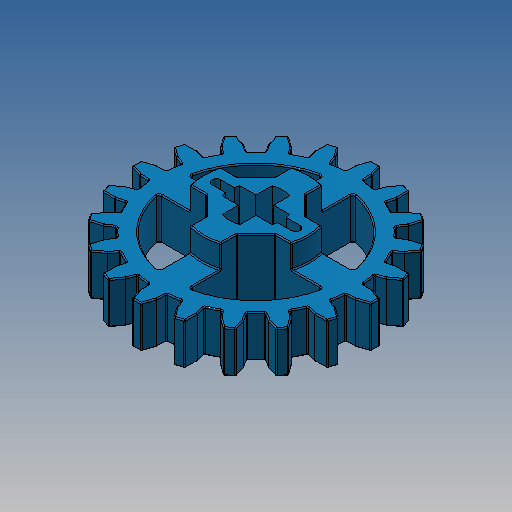
# Autodesk Inventor part: 69779-DkAzure
Saved by Autodesk Inventor 2025 (Build 290162010, 162A)
## iProperties
Created: 2014-08-13
Part Number: 69779-DkAzure
Material: ABS Plastic
Document SubType Name: Modeling
Designer: h.muther
Density: 1.06 g/cm^3
Appearance: DkAzure
Mass: 0.705537 g
Surface Area: 11.2279 cm^2
Volume: 0.665601 cm^3
Description: Technic, Gear 20
Author: h.muther
Autodesk Inventor part; units mm, degrees
ref_plane "YZ Plane" through (0, 0, 0) normal (1, 0, 0) x (0, 1, 0)
ref_plane "XZ Plane" through (0, 0, 0) normal (0, 1, 0) x (-1, 0, 0)
ref_plane "XY Plane" through (0, 0, 0) normal (0, 0, 1) x (1, 0, 0)
sketch "Sketch2" plane through (0, 0, 0) normal (0, 1, 0) x (-1, 0, 0)
  circle A0 centre (0, 0) radius 2.4 construction
  circle A1 centre (0, 0) radius 8.9654
  circle A2 centre (0, 0) radius 7.5654 construction
  circle A3 centre (0, 0) radius 4.8 construction
  circle A4 centre (0, 0) radius 3.6 construction
  line L0 (-0.8, 2.2627) -> (-0.8, 0.8)
  line L1 (-0.8, 0.8) -> (-2.2627, 0.8)
  line L2 (-2.2627, -0.8) -> (-0.8, -0.8)
  line L3 (-0.8, -0.8) -> (-0.8, -2.2627)
  line L4 (0.8, -2.2627) -> (0.8, -0.8)
  line L5 (0.8, -0.8) -> (2.2627, -0.8)
  line L6 (2.2627, 0.8) -> (0.8, 0.8)
  line L7 (0.8, 0.8) -> (0.8, 2.2627)
  arc A5 (0.8, 2.2627) -> (-0.8, 2.2627) centre (0, 0) ccw
  arc A6 (-2.2627, 0.8) -> (-2.2627, -0.8) centre (0, 0) ccw
  arc A7 (-0.8, -2.2627) -> (0.8, -2.2627) centre (0, 0) ccw
  arc A8 (2.2627, -0.8) -> (2.2627, 0.8) centre (0, 0) ccw
  line L8 (1.4, -7.4347) -> (1.4, -3.1255)
  line L9 (1.4, -3.1255) -> (3.1255, -1.4)
  line L10 (3.1255, -1.4) -> (7.4347, -1.4)
  line L11 (-3.6, 0.4) -> (-2.3664, 0.4)
  line L12 (-3.6, -0.4) -> (-2.3664, -0.4)
  arc A9 (-3.6, 0.4) -> (-3.6, -0.4) centre (-3.6, 0) ccw
  line L13 (2.3664, 0.4) -> (3.6, 0.4)
  arc A10 (3.6, -0.4) -> (3.6, 0.4) centre (3.6, 0) ccw
  line L14 (3.6, -0.4) -> (2.3664, -0.4)
  line L15 (-1.4, -7.4347) -> (-1.4, -3.1255)
  line L16 (-1.4, -3.1255) -> (-3.1255, -1.4)
  line L17 (-3.1255, -1.4) -> (-7.4347, -1.4)
  line L18 (-7.4347, 1.4) -> (-3.1255, 1.4)
  line L19 (-3.1255, 1.4) -> (-1.4, 3.1255)
  line L20 (-1.4, 3.1255) -> (-1.4, 7.4347)
  line L21 (1.4, 7.4347) -> (1.4, 3.1255)
  line L22 (1.4, 3.1255) -> (3.1255, 1.4)
  line L23 (3.1255, 1.4) -> (7.4347, 1.4)
  arc A11 (-7.4347, -1.4) -> (-1.4, -7.4347) centre (0, 0) ccw
  arc A12 (1.4, -7.4347) -> (7.4347, -1.4) centre (0, 0) ccw
  arc A13 (7.4347, 1.4) -> (1.4, 7.4347) centre (0, 0) ccw
  arc A14 (-1.4, 7.4347) -> (-7.4347, 1.4) centre (0, 0) ccw
  arc A15 (-1.4, -4.5913) -> (1.4, -4.5913) centre (0, 0) ccw
  arc A16 (4.5913, -1.4) -> (4.5913, 1.4) centre (0, 0) ccw
  arc A17 (-4.5913, 1.4) -> (-4.5913, -1.4) centre (0, 0) ccw
  arc A18 (1.4, 4.5913) -> (-1.4, 4.5913) centre (0, 0) ccw
  line L24 (-0.8, 8.9296) -> (-0.75, 9.7814)
  line L25 (-0.75, 9.7814) -> (-0.4, 10.8294)
  line L26 (-0.4, 10.8294) -> (0.4, 10.8294)
  line L27 (0.4, 10.8294) -> (0.75, 9.7814)
  line L28 (0.75, 9.7814) -> (0.8, 8.9296)
  point P0 (0, 10.8294)
  dimension "d1" = 4.8
  dimension "d9" = 9.6
  dimension "d2" = 1.6
  dimension "d3" = 0.8
  dimension "d4" = 7.2
  dimension "d6" = 135
  dimension "d7" = 2.8
  dimension "d8" = 6.4
  dimension "d10" = 10.8294
  dimension "d11" = 0.8
  dimension "d12" = 1.5
  dimension "d13" = 1.6
  dimension "d14" = 1.048
  dimension "d30" = 1.864
  dimension "d31" = 1.4
  constraints: 58 end point, 36 point on circle, 16 centre point, 16 equal length, 12 perpendicular, 8 parallel, 8 point on line, 5 coincident, 5 horizontal alignment, 4 tangent, 3 horizontal, 3 vertical alignment, 1 equal radius, 1 midpoint, 1 vertical, 46 other
  measures "d2" distance between parallel lines of L0 L7
  measures "d3" distance between parallel lines of L11 L12
  measures "d4" diameter of A4
  measures "d6" angle of L16 L15
  measures "d7" distance between parallel lines of L8 L15
  measures "d8" distance between parallel lines of L9 L19
  measures "d10" distance from line of L26 A12.centre
  measures "d11" distance of L25.end L26.end
  measures "d12" distance of L27.end L24.end
  measures "d13" distance of L28.end L24.start
  measures "d14" distance from line of L27.end L26
  measures "d30" distance edge to line of A1 L26
extrude "Extrusion1" add sketch "Sketch2" along normal mid plane 3.8 contours A1
extrude "Extrusion2" add sketch "Sketch2" along normal mid plane 8 contours A15 L15 L16 L17 A17 L18 L19 L20 A18 L21 L22 L23 A16 L10 L9 L8
extrude "Extrusion3" add sketch "Sketch2" along normal mid plane 3.8 contours A1 L24 L25 L26 L27 L28
fillet "Fillet1" radius 0.1 6 edges at (0.75, 0, 9.7814) (0.8, 0, 8.9296) (0.4, 0, 10.8294) (-0.4, 0, 10.8294) (-0.75, 0, 9.7814) (-0.8, 0, 8.9296)
pattern_circular "Circular Pattern1" count 20 over 360 about axis through (0, 0, 0) along (0, 1, 0) of "Extrusion3", "Fillet1"
fillet "Rundung3" radius 0.2 8 edges at (-1.4, 0, -7.4347) (-7.4347, 0, -1.4) (-7.4347, 0, 1.4) (-1.4, 0, 7.4347) (1.4, 0, 7.4347) (7.4347, 0, 1.4) (1.4, 0, -7.4347) (7.4347, 0, -1.4)
fillet "Fillet2" radius 0.1 346 edges at (-9.1709, 1.9, -2.1671) (-8.7679, 1.9, -1.9839) (-8.855, 1.9, -1.4025) (-8.9518, 1.9, -0.8227) (-9.3917, 1.9, -0.7729) (-10.2775, 1.9, -0.5843) (-10.8294, 1.9, 0) (-10.2775, 1.9, 0.5843) (-9.3917, 1.9, 0.7729) (-8.9518, 1.9, 0.8227) (-1.4025, 1.9, 8.855) (-8.855, 1.9, 1.4025) (-0.8227, 1.9, 8.9518) (-0.7729, 1.9, 9.3917) (-0.5843, 1.9, 10.2775) (0, 1.9, 10.8294) (0.5843, 1.9, 10.2775) (0.7729, 1.9, 9.3917) (0.8227, 1.9, 8.9518) (1.4025, 1.9, 8.855) (1.9839, 1.9, 8.7679) (2.1671, 1.9, 9.1709) (2.6202, 1.9, 9.955) (3.3465, 1.9, 10.2993) (3.7316, 1.9, 9.5939) (3.6372, 1.9, 8.6932) (3.5487, 1.9, 8.2595) (4.0702, 1.9, 7.9882) (4.5962, 1.9, 7.7257) (4.895, 1.9, 8.0523) (5.5682, 1.9, 8.6581) (6.3653, 1.9, 8.7611) (6.5137, 1.9, 7.9712) (6.1456, 1.9, 7.1438) (5.9273, 1.9, 6.7586) (6.3395, 1.9, 6.3395) (6.7586, 1.9, 5.9273) (7.1438, 1.9, 6.1456) (7.9712, 1.9, 6.5137) (8.7611, 1.9, 6.3653) (8.6581, 1.9, 5.5682) (8.0523, 1.9, 4.895) (7.7257, 1.9, 4.5962) (7.9882, 1.9, 4.0702) (8.2595, 1.9, 3.5487) (8.6932, 1.9, 3.6372) (9.5939, 1.9, 3.7316) (10.2993, 1.9, 3.3465) (9.955, 1.9, 2.6202) (9.1709, 1.9, 2.1671) (8.7679, 1.9, 1.9839) (8.855, 1.9, 1.4025) (8.9518, 1.9, 0.8227) (9.3917, 1.9, 0.7729) (10.2775, 1.9, 0.5843) (10.8294, 1.9, 0) (10.2775, 1.9, -0.5843) (9.3917, 1.9, -0.7729) (8.9518, 1.9, -0.8227) (8.855, 1.9, -1.4025) (8.7679, 1.9, -1.9839) (9.1709, 1.9, -2.1671) (9.955, 1.9, -2.6202) (10.2993, 1.9, -3.3465) (9.5939, 1.9, -3.7316) (8.6932, 1.9, -3.6372) (8.2595, 1.9, -3.5487) (7.9882, 1.9, -4.0702) (-7.7257, 1.9, -4.5962) (-7.9882, 1.9, -4.0702) (-8.2595, 1.9, -3.5487) (-8.6932, 1.9, -3.6372) (-9.5939, 1.9, -3.7316) (-10.2993, 1.9, -3.3465) (-9.955, 1.9, -2.6202) (-3.6372, 1.9, -8.6932) (-3.5487, 1.9, -8.2595) (-4.0702, 1.9, -7.9882) (-4.5962, 1.9, -7.7257) (-4.895, 1.9, -8.0523) (-5.5682, 1.9, -8.6581) (-6.3653, 1.9, -8.7611) (-6.5137, 1.9, -7.9712) (-6.1456, 1.9, -7.1438) (-5.9273, 1.9, -6.7586) (-6.3395, 1.9, -6.3395) (-6.7586, 1.9, -5.9273) (-7.1438, 1.9, -6.1456) (-7.9712, 1.9, -6.5137) (-8.7611, 1.9, -6.3653) (-8.6581, 1.9, -5.5682) (-8.0523, 1.9, -4.895) (0.5843, 1.9, -10.2775) (0, 1.9, -10.8294) (-0.5843, 1.9, -10.2775) (-0.7729, 1.9, -9.3917) (-0.8227, 1.9, -8.9518) (-1.4025, 1.9, -8.855) (-1.9839, 1.9, -8.7679) (-2.1671, 1.9, -9.1709) (-2.6202, 1.9, -9.955) (-3.3465, 1.9, -10.2993) (-3.7316, 1.9, -9.5939) (7.7257, 1.9, -4.5962) (8.0523, 1.9, -4.895) (8.6581, 1.9, -5.5682) (8.7611, 1.9, -6.3653) (7.9712, 1.9, -6.5137) (7.1438, 1.9, -6.1456) (6.7586, 1.9, -5.9273) (6.3395, 1.9, -6.3395) (5.9273, 1.9, -6.7586) (6.1456, 1.9, -7.1438) (6.5137, 1.9, -7.9712) (6.3653, 1.9, -8.7611) (5.5682, 1.9, -8.6581) (4.895, 1.9, -8.0523) (4.5962, 1.9, -7.7257) (4.0702, 1.9, -7.9882) (3.5487, 1.9, -8.2595) (3.6372, 1.9, -8.6932) (3.7316, 1.9, -9.5939) (3.3465, 1.9, -10.2993) (2.6202, 1.9, -9.955) (2.1671, 1.9, -9.1709) (1.9839, 1.9, -8.7679) (1.4025, 1.9, -8.855) (0.8227, 1.9, -8.9518) (0.7729, 1.9, -9.3917) (0, 4, 4.8) (1.4, 2.95, 4.5913) (1.4, 1.9, 5.8904) (-1.4, 1.9, 5.8904) (-1.4, 2.95, 4.5913) (0, 1.9, 4.8) (-5.3495, 1.9, 5.3495) (-5.8904, 1.9, 1.4) (-4.5913, 2.95, 1.4) (-3.8584, 4, 1.4) (-2.2627, 4, 2.2627) (-1.4, 4, 3.8584) (1.4, 4, 3.8584) (1.4, 0, 3.1255) (2.2627, 4, 2.2627) (3.1255, 0, 1.4) (3.8584, 4, 1.4) (4.5913, 2.95, 1.4) (5.8904, 1.9, 1.4) (5.3495, 1.9, 5.3495) (4.8, 1.9, 0) (4.8, 4, 0) (4.5913, 2.95, -1.4) (5.8904, 1.9, -1.4) (5.3495, 1.9, -5.3495) (1.4, 1.9, -5.8904) (3.1255, 0, -1.4) (1.4, 0, -3.1255) (3.8584, 4, -1.4) (2.2627, 4, -2.2627) (1.4, 4, -3.8584) (1.4, 2.95, -4.5913) (0, 4, -4.8) (-1.4, 2.95, -4.5913) (0, 1.9, -4.8) (-1.4, 1.9, -5.8904) (-5.3495, 1.9, -5.3495) (-5.8904, 1.9, -1.4) (-4.5913, 2.95, -1.4) (-4.8, 4, 0) (-3.8584, 4, -1.4) (-2.2627, 4, -2.2627) (-1.4, 4, -3.8584) (-1.4, 0, -3.1255) (-3.1255, 0, -1.4) (-3.1255, 0, 1.4) (-1.4, 0, 3.1255) (-4.8, 1.9, 0) (-6.5137, -1.9, -7.9712) (-6.3653, -1.9, -8.7611) (-5.5682, -1.9, -8.6581) (-4.895, -1.9, -8.0523) (-4.5962, -1.9, -7.7257) (-4.0702, -1.9, -7.9882) (-3.5487, -1.9, -8.2595) (-3.6372, -1.9, -8.6932) (-3.7316, -1.9, -9.5939) (-3.3465, -1.9, -10.2993) (-2.6202, -1.9, -9.955) (-2.1671, -1.9, -9.1709) (-1.9839, -1.9, -8.7679) (-1.4025, -1.9, -8.855) (-0.8227, -1.9, -8.9518) (-0.7729, -1.9, -9.3917) (-0.5843, -1.9, -10.2775) (0, -1.9, -10.8294) (0.5843, -1.9, -10.2775) (0.7729, -1.9, -9.3917) (0.8227, -1.9, -8.9518) (1.4025, -1.9, -8.855) (1.9839, -1.9, -8.7679) (2.1671, -1.9, -9.1709) (2.6202, -1.9, -9.955) (3.3465, -1.9, -10.2993) (3.7316, -1.9, -9.5939) (3.6372, -1.9, -8.6932) (3.5487, -1.9, -8.2595) (4.0702, -1.9, -7.9882) (4.5962, -1.9, -7.7257) (4.895, -1.9, -8.0523) (5.5682, -1.9, -8.6581) (6.3653, -1.9, -8.7611) (6.5137, -1.9, -7.9712) (6.1456, -1.9, -7.1438) (5.9273, -1.9, -6.7586) (6.3395, -1.9, -6.3395) (6.7586, -1.9, -5.9273) (7.1438, -1.9, -6.1456) (7.9712, -1.9, -6.5137) (8.7611, -1.9, -6.3653) (8.6581, -1.9, -5.5682) (8.0523, -1.9, -4.895) (7.7257, -1.9, -4.5962) (7.9882, -1.9, -4.0702) (8.2595, -1.9, -3.5487) (8.6932, -1.9, -3.6372) (9.5939, -1.9, -3.7316) (10.2993, -1.9, -3.3465) (9.955, -1.9, -2.6202) (9.1709, -1.9, -2.1671) (8.7679, -1.9, -1.9839) (8.855, -1.9, -1.4025) (8.9518, -1.9, -0.8227) (9.3917, -1.9, -0.7729) (10.2775, -1.9, -0.5843) (10.8294, -1.9, 0) (10.2775, -1.9, 0.5843) (9.3917, -1.9, 0.7729) (8.9518, -1.9, 0.8227) (8.855, -1.9, 1.4025) (8.7679, -1.9, 1.9839) (9.1709, -1.9, 2.1671) (9.955, -1.9, 2.6202) (10.2993, -1.9, 3.3465) (-0.7729, -1.9, 9.3917) (-0.5843, -1.9, 10.2775) (0, -1.9, 10.8294) (0.5843, -1.9, 10.2775) (0.7729, -1.9, 9.3917) (0.8227, -1.9, 8.9518) (1.4025, -1.9, 8.855) (1.9839, -1.9, 8.7679) (2.1671, -1.9, 9.1709) (2.6202, -1.9, 9.955) (3.3465, -1.9, 10.2993) (3.7316, -1.9, 9.5939) (3.6372, -1.9, 8.6932) (3.5487, -1.9, 8.2595) (4.0702, -1.9, 7.9882) (4.5962, -1.9, 7.7257) (4.895, -1.9, 8.0523) (5.5682, -1.9, 8.6581) (6.3653, -1.9, 8.7611) (6.5137, -1.9, 7.9712) (6.1456, -1.9, 7.1438) (5.9273, -1.9, 6.7586) (6.3395, -1.9, 6.3395) (6.7586, -1.9, 5.9273) (7.1438, -1.9, 6.1456) (7.9712, -1.9, 6.5137) (8.7611, -1.9, 6.3653) (8.6581, -1.9, 5.5682) (8.0523, -1.9, 4.895) (7.7257, -1.9, 4.5962) (7.9882, -1.9, 4.0702) (8.2595, -1.9, 3.5487) (8.6932, -1.9, 3.6372) (9.5939, -1.9, 3.7316) (-10.2775, -1.9, 0.5843) (-10.8294, -1.9, 0) (-10.2775, -1.9, -0.5843) (-9.3917, -1.9, -0.7729) (-8.9518, -1.9, -0.8227) (-8.855, -1.9, -1.4025) (-8.7679, -1.9, -1.9839) (-9.1709, -1.9, -2.1671) (-9.955, -1.9, -2.6202) (-10.2993, -1.9, -3.3465) (-9.5939, -1.9, -3.7316) (-8.6932, -1.9, -3.6372) (-8.2595, -1.9, -3.5487) (-7.9882, -1.9, -4.0702) (-7.7257, -1.9, -4.5962) (-8.0523, -1.9, -4.895) (-8.6581, -1.9, -5.5682) (-8.7611, -1.9, -6.3653) (-7.9712, -1.9, -6.5137) (-7.1438, -1.9, -6.1456) (-6.7586, -1.9, -5.9273) (-6.3395, -1.9, -6.3395) (-5.9273, -1.9, -6.7586) (-6.1456, -1.9, -7.1438) (-0.8227, -1.9, 8.9518) (-1.4025, -1.9, 8.855) (-8.855, -1.9, 1.4025) (-8.9518, -1.9, 0.8227) (-9.3917, -1.9, 0.7729) (-1.4, -2.95, 4.5913) (-1.4, -1.9, 5.8904) (-5.3495, -1.9, 5.3495) (-5.8904, -1.9, 1.4) (-4.8, -1.9, 0) (-4.5913, -2.95, 1.4) (-4.8, -4, 0) (-3.8584, -4, 1.4) (-2.2627, -4, 2.2627) (-1.4, -4, 3.8584) (0, -1.9, 4.8) (0, -4, 4.8) (1.4, -2.95, 4.5913) (1.4, -4, 3.8584) (2.2627, -4, 2.2627) (1.4, -1.9, 5.8904) (5.3495, -1.9, 5.3495) (4.5913, -2.95, 1.4) (5.8904, -1.9, 1.4) (3.8584, -4, 1.4) (4.8, -4, 0) (3.8584, -4, -1.4) (4.5913, -2.95, -1.4) (4.8, -1.9, 0) (5.8904, -1.9, -1.4) (5.3495, -1.9, -5.3495) (2.2627, -4, -2.2627) (1.4, -4, -3.8584) (1.4, -2.95, -4.5913) (0, -4, -4.8) (1.4, -1.9, -5.8904) (-1.4, -1.9, -5.8904) (0, -1.9, -4.8) (-1.4, -2.95, -4.5913) (-1.4, -4, -3.8584) (-5.3495, -1.9, -5.3495) (-5.8904, -1.9, -1.4) (-4.5913, -2.95, -1.4) (-3.8584, -4, -1.4) (-2.2627, -4, -2.2627)
equation "\"d1\" = kd"
equation "\"d2\" = axlet"
equation "\"d17\" = lu"
equation "\"kd\" = 4.8"
equation "\"axlet\" = 1.6"
equation "\"lu\" = 8"
body "Solid1"
